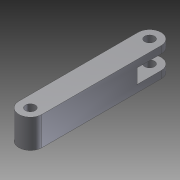
# Autodesk Inventor part: F
Saved by Autodesk Inventor 2011 SP2 (Build 150309200, 309)
## iProperties
Created: 2014-05-09
Part Number: F
Document SubType Name: Modeling
Designer: Maurice Woods
Density: 1 g/cm^3
Author: Maurice Woods
Autodesk Inventor part; units mm, degrees
ref_plane "YZ Plane" through (0, 0, 0) normal (1, 0, 0) x (0, 1, 0)
ref_plane "XZ Plane" through (0, 0, 0) normal (0, 1, 0) x (-1, 0, 0)
ref_plane "XY Plane" through (0, 0, 0) normal (0, 0, 1) x (1, 0, 0)
sketch "Sketch1" plane through (0, 0, 0) normal (0, 0, 1) x (1, 0, 0)
  line L0 (0, 24.6876) -> (0, 24.6876)
  line L1 (4, 20.6876) -> (4, 12.3438)
  line L2 (0, -24.6876) -> (0, -24.6876)
  line L3 (-4, -20.6876) -> (-4, -11.5899)
  line L4 (-4, 24.6876) -> (0, 24.6876) construction
  line L5 (0, 24.6876) -> (0, 0) construction
  line L6 (0, 0) -> (-4, 0) construction
  line L7 (-4, 0) -> (-4, 24.6876) construction
  arc A0 (4, 20.6876) -> (0, 24.6876) centre (0, 20.6876) ccw
  arc A1 (0, 24.6876) -> (-4, 20.6876) centre (0, 20.6876) ccw
  arc A2 (-4, -20.6876) -> (0, -24.6876) centre (0, -20.6876) ccw
  arc A3 (0, -24.6876) -> (4, -20.6876) centre (0, -20.6876) ccw
  line L8 (-4, 5.437) -> (4, 12.3438)
  line L9 (-4, 5.437) -> (-4, 20.6876)
  line L10 (4, 12.3438) -> (4, -13.4441)
  line L11 (-4, -11.5899) -> (4, -13.4441)
  line L12 (-4, -11.5899) -> (-4, 5.437)
  line L13 (4, -13.4441) -> (4, -20.6876)
  dimension "d0" = 4
  dimension "d6" = 41.3753
  constraints: 28 end point, 16 tangent, 12 parallel, 8 point on circle, 4 centre point, 4 perpendicular, 3 equal radius, 2 coincident, 2 horizontal, 2 point on line, 2 other
  measures "d0" radius of A0
  measures "d6" distance of A2.centre A0.centre
extrude "Extrusion5" add sketch "Sketch1" along normal mid plane 10
extrude "Extrusion6" cut sketch "Sketch1" along normal mid plane 5 contours L1 L8 L9 A1 A0 | L13 A3 A2 L3 L11
sketch "Sketch4" plane through (0, 0, 5) normal (0, 0, 1) x (1, 0, 0)
  arc A0 (4, 20.6876) -> (-4, 20.6876) centre (0, 20.6876) ccw projected
  arc A1 (-4, -20.6876) -> (4, -20.6876) centre (0, -20.6876) ccw projected
  point P0 (0, 0)
hole "Hole3" at (0, -20.6876, 5) at (0, 20.6876, 5) direction (0, 0, -1) diameter 3.4 end through all
fillet "Fillet1" radius 2 4 edges at (4, -13.4441, 0) (4, 12.3438, 0) (-4, 5.437, 0) (-4, -11.5899, 0)
equation "\"d6\" = LengthK"
equation "\"LengthK\" = 41.375254"
body "Solid4"
